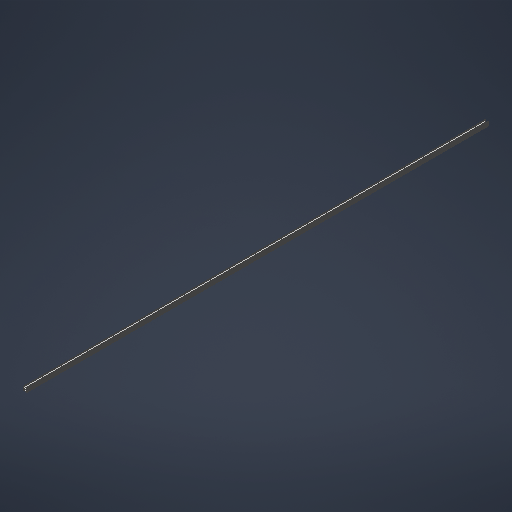
# Autodesk Inventor part: SP40-09 MARCO CORREDERA
Saved by Autodesk Inventor 2025 (Build 290162000, 162)
## iProperties
Created: 2026-01-17
Part Number: SP40-09 MARCO CORREDERA
Material: Aluminio
Document SubType Name: Modeling
Designer: ROLANDO
Density: 2.7 g/cm^3
Appearance: Satinado
Author: ROLANDO
Autodesk Inventor part; units mm, degrees
ref_plane "YZ Plane" through (0, 0, 0) normal (1, 0, 0) x (0, 1, 0)
ref_plane "XZ Plane" through (0, 0, 0) normal (0, 1, 0) x (-1, 0, 0)
ref_plane "XY Plane" through (0, 0, 0) normal (0, 0, 1) x (1, 0, 0)
sketch "Boceto1" plane through (0, 0, 0) normal (0, 0, 1) x (1, 0, 0)
  line L0 (-31.1865, 21.1784) -> (-31.1865, 0.1784)
  line L1 (-29.2865, 4.1784) -> (11.9135, 4.1784)
  line L2 (13.8135, 0.1784) -> (13.8135, 15.7784)
  line L3 (6.7135, 42.7016) -> (6.7135, 21.1784)
  line L4 (-29.7865, 19.7784) -> (8.4135, 19.7784)
  line L5 (12.4135, 15.7784) -> (12.4135, 6.0784)
  line L6 (11.9135, 5.5784) -> (-29.2865, 5.5784)
  line L7 (-29.7865, 6.0784) -> (-29.7865, 19.7784)
  arc A0 (12.4135, 15.7784) -> (8.4135, 19.7784) centre (8.4135, 15.7784) ccw
  line L8 (12.4135, 3.6784) -> (12.4135, 1.9253)
  line L9 (11.3135, 0.1784) -> (13.8135, 0.1784)
  line L10 (5.3135, 21.1784) -> (5.3135, 43.8878)
  line L11 (-29.7865, 3.6784) -> (-29.7865, 1.8562)
  line L12 (-28.6865, 0.1784) -> (-31.1865, 0.1784)
  line L13 (-28.6865, 0.1784) -> (-28.6865, 0.6338)
  line L14 (11.3135, 0.1784) -> (11.3135, 0.8784)
  line L15 (-28.9312, 1.0637) -> (-29.5418, 1.4262)
  line L16 (11.3135, 0.8784) -> (12.2053, 1.5192)
  arc A1 (11.9135, 5.5784) -> (12.4135, 6.0784) centre (11.9135, 6.0784) ccw
  arc A2 (12.4135, 3.6784) -> (11.9135, 4.1784) centre (11.9135, 3.6784) ccw
  arc A3 (12.2053, 1.5192) -> (12.4135, 1.9253) centre (11.9135, 1.9253) ccw
  arc A4 (-29.7865, 6.0784) -> (-29.2865, 5.5784) centre (-29.2865, 6.0784) ccw
  arc A5 (-29.2865, 4.1784) -> (-29.7865, 3.6784) centre (-29.2865, 3.6784) ccw
  arc A6 (-29.7865, 1.8562) -> (-29.5418, 1.4262) centre (-29.2865, 1.8562) ccw
  arc A7 (-28.6865, 0.6338) -> (-28.9312, 1.0637) centre (-29.1865, 0.6338) ccw
  line L17 (5.3135, 43.8878) -> (10.0635, 44.6784)
  line L18 (10.0635, 44.6784) -> (14.8135, 43.8878)
  line L19 (6.7135, 42.7016) -> (10.0635, 43.2591)
  line L20 (10.0635, 43.2591) -> (13.4135, 42.7016)
  line L21 (14.8135, 43.8878) -> (14.8135, 36.0884)
  line L22 (14.8135, 36.0884) -> (13.4135, 36.0884)
  line L23 (13.4135, 36.0884) -> (13.4135, 42.7016)
  line L24 (6.7135, 21.1784) -> (8.4135, 21.1784)
  arc A8 (13.8135, 15.7784) -> (8.4135, 21.1784) centre (8.4135, 15.7784) ccw
  line L25 (10.0635, 52.6138) -> (10.0635, 36.0884) construction
  line L26 (-24.0865, 42.7016) -> (-24.0865, 21.1784)
  line L27 (-22.6865, 21.1784) -> (-22.6865, 43.8878)
  line L28 (-22.6865, 43.8878) -> (-27.4365, 44.6784)
  line L29 (-27.4365, 44.6784) -> (-32.1865, 43.8878)
  line L30 (-24.0865, 42.7016) -> (-27.4365, 43.2591)
  line L31 (-27.4365, 43.2591) -> (-30.7865, 42.7016)
  line L32 (-32.1865, 43.8878) -> (-32.1865, 36.0884)
  line L33 (-32.1865, 36.0884) -> (-30.7865, 36.0884)
  line L34 (-30.7865, 36.0884) -> (-30.7865, 42.7016)
  line L35 (-27.4365, 52.6138) -> (-27.4365, 36.0884) construction
  line L36 (5.3135, 21.1784) -> (-22.6865, 21.1784)
  line L37 (-24.0865, 21.1784) -> (-31.1865, 21.1784)
  line L38 (-8.6865, 50.2757) -> (-8.6865, -0.697) construction
  point P0 (0, 0)
  point P1 (-29.7865, 1.5715)
  point P2 (-28.6865, 0.9184)
  dimension "d17" = 4
  dimension "d24" = 1.4
  dimension "d50" = 0.7
  dimension "d61" = 0.74
  dimension "d62" = 30.7
  dimension "d63" = 35.7
  dimension "d206" = 1.4
  dimension "d207" = 1.4
  dimension "d210" = 1.4
  dimension "d211" = 1.4
  dimension "d213" = 14.2
  dimension "d214" = 1.4
  dimension "d215" = 1.4
  dimension "d216" = 1.4
  dimension "d217" = 1.4
  dimension "d218" = 45
  dimension "d223" = 5.4
  dimension "d224" = 1.4
  dimension "d225" = 9.5
  dimension "d226" = 4.75
  dimension "d227" = 3.35
  dimension "d228" = 6.7
  dimension "d229" = 44.5
  dimension "d230" = 3.35
  dimension "d231" = 2.5
  dimension "d232" = 2.5
  dimension "d240" = 8.59
  dimension "d241" = 3.35
  dimension "d242" = 99.45
  dimension "d243" = 161.1
  dimension "d246" = 1.4
  dimension "d247" = 1.4
  dimension "d248" = 1.4
  dimension "d253" = 1.4
  dimension "d254" = 1.4
  dimension "d255" = 1.4
  dimension "d256" = 1.4
  dimension "d257" = 8.59
  dimension "d258" = 161.1
  dimension "d259" = 99.45
  dimension "d260" = 22.5
  dimension "d266" = 23.5
  dimension "d267" = 47
  dimension "d268" = 3.35
  dimension "d269" = 9.5
  dimension "d270" = 4.75
  dimension "d271" = 3.35
  dimension "d272" = 6.7
  dimension "d273" = 28
  dimension "d274" = 37.5
  dimension "d275" = 8.5
  dimension "d276" = 8.5
  dimension "d277" = 44.5
  dimension "d278" = 0.5
  dimension "d279" = 14.91
  dimension "d280" = 14.91
  dimension "d281" = 14.8135
  dimension "d282" = 36.0884
  dimension "d283" = 16.5254
  dimension "d284" = 0
  dimension "d285" = 14.1873
  dimension "d286" = 36.7854
  dimension "d287" = 16.5254
  dimension "d288" = 0
  constraints: 78 end point, 18 point on circle, 18 tangent, 10 parallel, 9 centre point, 6 equal radius, 6 point on line, 5 collinear, 5 perpendicular, 4 horizontal, 2 vertical
  measures "d17" radius of A0
  measures "d24" distance between parallel lines of L1 L6
  measures "d50" distance of L9.start L14.end
  measures "d61" distance of L12.start point (-28.686, 0.918)
  measures "d62" angle of L12 L15
  measures "d63" angle of L9 L16
  measures "d206" distance between parallel lines of L21 L23
  measures "d207" distance between parallel lines of L3 L10
  measures "d210" distance between parallel lines of L17 L19
  measures "d211" distance between parallel lines of L18 L20
  measures "d213" distance between parallel lines of L4 L6
  measures "d214" distance between parallel lines of L8 L2
  measures "d215" distance between parallel lines of L2 L5
  measures "d216" distance between parallel lines of L0 L7
  measures "d217" distance between parallel lines of L0 L11
  measures "d218" distance between parallel lines of L2 L0
  measures "d223" radius of A8
  measures "d224" radial gap between concentric circles of A8 A0
  measures "d225" distance between parallel lines of L21 L10
  measures "d226" distance from line of L10 L17.end
  measures "d227" distance from line of L3 L19.end
  measures "d228" distance between parallel lines of L23 L3
  measures "d229" distance from line of L9 L17.end
  measures "d230" horizontal distance of L19.end L20.end
  measures "d231" distance of L9.start L2.start
  measures "d232" distance of L12.start L0.end
  measures "d240" distance from line of L17.end L22
  measures "d241" distance between parallel lines of L3 L25
  measures "d242" angle of L25 L18
  measures "d243" angle of L17 L18
  measures "d246" distance between parallel lines of L4 L37
  measures "d247" distance between parallel lines of L4 L36
  measures "d248" distance between parallel lines of L4 L24
  measures "d253" distance between parallel lines of L26 L27
  measures "d254" distance between parallel lines of L28 L30
  measures "d255" distance between parallel lines of L29 L31
  measures "d256" distance between parallel lines of L32 L34
  measures "d257" distance from line of L28.end L33
  measures "d258" angle of L29 L28
  measures "d259" angle of L35 L29
  measures "d260" distance between parallel lines of L2 L38
  measures "d266" distance between parallel lines of L38 L21
  measures "d267" distance between parallel lines of L21 L32
  measures "d268" distance between parallel lines of L26 L35
  measures "d269" distance between parallel lines of L32 L27
  measures "d270" distance between parallel lines of L35 L27
  measures "d271" distance between parallel lines of L34 L35
  measures "d272" distance between parallel lines of L26 L34
  measures "d273" distance between parallel lines of L10 L27
  measures "d274" distance between parallel lines of L25 L35
  measures "d275" distance between parallel lines of L0 L27
  measures "d276" distance between parallel lines of L2 L10
  measures "d277" distance from line of L12 L28.end
  measures "d278" radius of A1
  measures "d279" distance between parallel lines of L36 L22
  measures "d280" distance between parallel lines of L37 L22
  measures "d281" distance from line of point (0, 0) L21
  measures "d282" distance from line of point (0, 0) L22
  measures "d283" distance from line of L25.start L22
  measures "d284" distance from line of L25.end L22
  measures "d285" distance from line of L38.start L22
  measures "d286" distance from line of L38.end L22
  measures "d287" distance from line of L35.start L22
  measures "d288" distance from line of L35.end L22
extrude "Extrusión1" add sketch "Boceto1" against normal blind 5800
